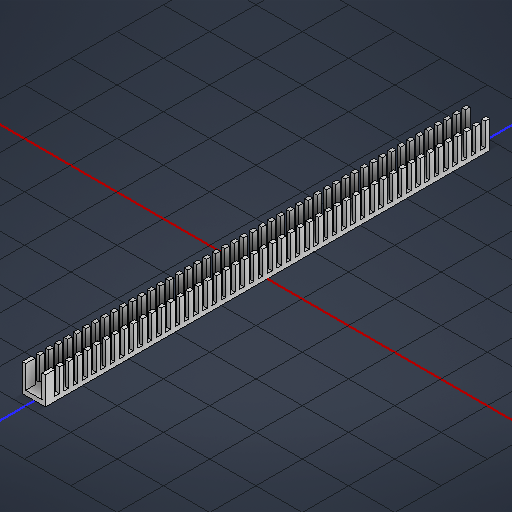
# Autodesk Inventor part: 000.005.002 - Кабель канал
Saved by Autodesk Inventor 2025 (Build 290162000, 162)
## iProperties
Created: 2024-08-11
Part Number: 000.005.002 - Кабель канал
Material: Типовые
Document SubType Name: Modeling
Designer: IvanPetrov
Density: 1 g/cm^3
Appearance: По умолчанию
Author: IvanPetrov
Autodesk Inventor part; units mm, degrees
ref_plane "YZ Plane" through (0, 0, 0) normal (1, 0, 0) x (0, 1, 0)
ref_plane "XZ Plane" through (0, 0, 0) normal (0, 1, 0) x (-1, 0, 0)
ref_plane "XY Plane" through (0, 0, 0) normal (0, 0, 1) x (1, 0, 0)
sketch "Эскиз1" plane through (0, 0, 0) normal (0, 1, 0) x (-1, 0, 0)
  line L0 (-5, 96) -> (5, 96)
  line L1 (5, 96) -> (5, -96)
  line L2 (5, -96) -> (-5, -96)
  line L3 (-5, -96) -> (-5, 96)
  line L4 (-5, 96) -> (5, -96) construction
  line L5 (5, 96) -> (-5, -96) construction
  point P0 (0, 0)
  dimension "d0" = 10
  dimension "d1" = 192
  constraints: 12 end point, 2 midpoint, 2 parallel, 1 horizontal, 1 perpendicular
  measures "d0" distance of L1.end L2.end
  measures "d1" distance of L0.end L1.end
extrude "Выдавливание1" add sketch "Эскиз1" along normal blind 2
sketch "Эскиз2" plane through (0, 2, 0) normal (0, 1, 0) x (1, 0, 0)
  line L0 (-5, 96) -> (-5, -96) projected
  line L1 (5, -96) -> (-5, -96)
  line L2 (-5, -96) -> (-5, 96)
  line L3 (-5, 96) -> (5, 96)
  line L4 (5, 96) -> (5, -96)
  line L5 (5, -96) -> (-5, 96) construction
  line L6 (-5, -96) -> (5, 96) construction
  line L7 (5, 96) -> (-5, 96) projected
  line L8 (3.5, -96) -> (-3.5, -96)
  line L9 (-3.5, -96) -> (-3.5, 96)
  line L10 (-3.5, 96) -> (3.5, 96)
  line L11 (3.5, 96) -> (3.5, -96)
  line L12 (3.5, -96) -> (-3.5, 96) construction
  line L13 (-3.5, -96) -> (3.5, 96) construction
  point P0 (0, 0)
  dimension "d4" = 1.5
  constraints: 24 end point, 4 midpoint, 4 parallel, 2 horizontal, 2 perpendicular, 1 point on line
  measures "d4" distance between parallel lines of L0 L9
extrude "Выдавливание2" add sketch "Эскиз2" along normal blind 10 contours L3 L9 L1 L0 | L3 L4 L1 L11
sketch "Эскиз3" plane through (0, 12, 0) normal (0, 1, 0) x (1, 0, 0)
  line L0 (-5, 96) -> (-5, -96) projected
  line L1 (-5, 94) -> (5, 94)
  line L2 (5, 94) -> (5, 92)
  line L3 (5, 92) -> (-5, 92)
  line L4 (-5, 92) -> (-5, 94)
  line L5 (3.5, 96) -> (-3.5, 96) projected
  point P0 (0, 0)
  dimension "d7" = 2
  dimension "d8" = 2
  constraints: 8 end point, 2 parallel, 1 horizontal, 1 perpendicular, 1 point on line
  measures "d7" distance between parallel lines of L1 L3
  measures "d8" distance between parallel lines of L5 L1
extrude "Выдавливание3" cut sketch "Эскиз3" against normal up to surface (10 mm away)
pattern_linear "Прямоуг.массив1" count 47 spacing 4 along (0, 0, 1) of "Выдавливание3"
